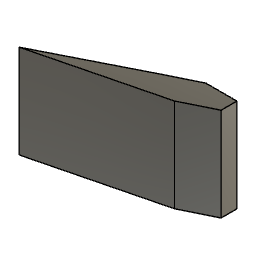
Stabalising scoop v5 (Autodesk Fusion 360 design; units mm, degrees)
Autodesk Fusion 360 part; units mm, degrees
sketch "Sketch4" plane through (0, 0, 0) normal (0, 0, 1) x (1, 0, 0)
  line L0 (0, 0) -> (30, 0)
  line L1 (30, 0) -> (30, 10)
  line L2 (30, 10) -> (0, 10)
  line L3 (0, 10) -> (0, 0)
  constraint horizontal L0
  constraint vertical L1
  constraint horizontal L2
  constraint vertical L3
  constraint coincident L0.start L3.end
sketch "Sketch5" plane through (0, 0, 0) normal (0, 0, 1) x (1, 0, 0)
  line L0 (0, 0) -> (20, 5)
  line L1 (20, 5) -> (25.0128, 7.4566)
  line L2 (25.0128, 7.4566) -> (25.0128, 10)
  line L3 (25.0128, 10) -> (20, 10)
  line L4 (20, 10) -> (14.8103, 7.4566)
  line L5 (14.8103, 7.4566) -> (0, 0)
  constraint coincident L0.start L5.end
  constraint vertical L2
  constraint perpendicular L2 L3
  constraint parallel L1 L4
extrude "Extrude9" add sketch "Sketch5" along normal blind 15
